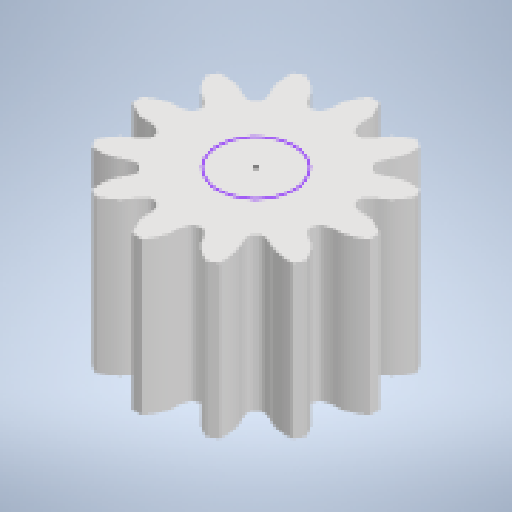
# Autodesk Inventor part: gear_3
Saved by Autodesk Inventor 2025.2 (Build 292293000, 293)
## iProperties
Created: 2025-03-25
Part Number: gear_3
Material: Generic
Document SubType Name: Modeling
Designer: Admin
Density: 1 g/cm^3
Appearance: Default
Author: Admin
Autodesk Inventor part; units mm, degrees
ref_plane "YZ Plane" through (0, 0, 0) normal (1, 0, 0) x (0, 1, 0)
ref_plane "XZ Plane" through (0, 0, 0) normal (0, 1, 0) x (-1, 0, 0)
ref_plane "XY Plane" through (0, 0, 0) normal (0, 0, 1) x (1, 0, 0)
sketch "Sketch1" plane through (0, 0, 0) normal (0, 1, 0) x (-1, 0, 0)
  arc A0 (0.3103, 6.9931) -> (-0.3103, 6.9931) centre (0, 0) ccw
  spline S0 degree 3 poles (-0.3103, 6.9931) (-0.3386, 6.9508) (-0.3937, 6.8652) (-0.4712, 6.7337) (-0.5433, 6.5992) (-0.6093, 6.4615) (-0.6693, 6.3211) (-0.7218, 6.1777) (-0.7653, 6.0313) (-0.7979, 5.8823) (-0.8227, 5.7311) (-0.8192, 5.5783) (-0.8156, 5.4255) (-0.8404, 5.2744) (-0.873, 5.1254) (-0.906, 5.0145) (-0.9268, 4.9533) (-0.9314, 4.9403) knots 0.009806 0.009806 0.009806 0.009806 0.07852 0.147233 0.215945 0.284657 0.353368 0.422077 0.490783 0.559487 0.628183 0.696834 0.765485 0.834181 0.902886 0.971592 0.990196 0.990196 0.990196 0.990196
  arc A1 (-1.2026, 4.6913) -> (-0.9314, 4.9403) centre (-1.2995, 5.0691) ccw
  arc A2 (-1.2026, 4.6913) -> (-1.3041, 4.6641) centre (0, 0) ccw
  arc A3 (-1.6636, 4.7441) -> (-1.3041, 4.6641) centre (-1.4091, 5.0397) ccw
  spline S1 degree 3 poles (-1.6636, 4.7441) (-1.674, 4.7531) (-1.7227, 4.7957) (-1.8066, 4.8752) (-1.9094, 4.988) (-2.0064, 5.1065) (-2.0798, 5.2406) (-2.1531, 5.3747) (-2.2501, 5.4932) (-2.3529, 5.6059) (-2.4638, 5.711) (-2.5809, 5.8089) (-2.7031, 5.9005) (-2.8291, 5.9867) (-2.9588, 6.0672) (-3.0917, 6.1423) (-3.1821, 6.1889) (-3.2278, 6.2114) knots 0.009805 0.009805 0.009805 0.009805 0.028409 0.097115 0.165819 0.234515 0.303166 0.371817 0.440513 0.509218 0.577924 0.646632 0.715343 0.784055 0.852768 0.921481 0.990194 0.990194 0.990194 0.990194
  arc A4 (-3.2278, 6.2114) -> (-3.7653, 5.901) centre (0, 0) ccw
  spline S2 degree 3 poles (-3.7653, 5.901) (-3.7687, 5.8503) (-3.7736, 5.7486) (-3.775, 5.596) (-3.7701, 5.4434) (-3.7584, 5.2912) (-3.7401, 5.1396) (-3.7139, 4.9892) (-3.6784, 4.8406) (-3.6322, 4.6952) (-3.578, 4.552) (-3.4986, 4.4214) (-3.4191, 4.2908) (-3.365, 4.1476) (-3.3188, 4.0022) (-3.2919, 3.8897) (-3.2793, 3.8263) (-3.2767, 3.8128) knots 0.009806 0.009806 0.009806 0.009806 0.07852 0.147233 0.215945 0.284657 0.353368 0.422077 0.490783 0.559487 0.628183 0.696834 0.765485 0.834181 0.902886 0.971592 0.990196 0.990196 0.990196 0.990196
  arc A5 (-3.3872, 3.4615) -> (-3.2767, 3.8128) centre (-3.6599, 3.7402) ccw
  arc A6 (-3.3872, 3.4615) -> (-3.4615, 3.3872) centre (0, 0) ccw
  arc A7 (-3.8128, 3.2767) -> (-3.4615, 3.3872) centre (-3.7402, 3.6599) ccw
  spline S3 degree 3 poles (-3.8128, 3.2767) (-3.8263, 3.2793) (-3.8897, 3.2919) (-4.0022, 3.3188) (-4.1476, 3.365) (-4.2908, 3.4191) (-4.4214, 3.4986) (-4.552, 3.578) (-4.6952, 3.6322) (-4.8406, 3.6784) (-4.9892, 3.7139) (-5.1396, 3.7401) (-5.2912, 3.7584) (-5.4434, 3.7701) (-5.596, 3.775) (-5.7486, 3.7736) (-5.8503, 3.7687) (-5.901, 3.7653) knots 0.009805 0.009805 0.009805 0.009805 0.028409 0.097115 0.165819 0.234515 0.303166 0.371817 0.440513 0.509218 0.577924 0.646632 0.715343 0.784055 0.852768 0.921481 0.990194 0.990194 0.990194 0.990194
  arc A8 (-5.901, 3.7653) -> (-6.2114, 3.2278) centre (0, 0) ccw
  spline S4 degree 3 poles (-6.2114, 3.2278) (-6.1889, 3.1821) (-6.1423, 3.0917) (-6.0672, 2.9588) (-5.9867, 2.8291) (-5.9005, 2.7031) (-5.8089, 2.5809) (-5.711, 2.4638) (-5.6059, 2.3529) (-5.4932, 2.2501) (-5.3747, 2.1531) (-5.2406, 2.0798) (-5.1065, 2.0064) (-4.988, 1.9094) (-4.8752, 1.8066) (-4.7957, 1.7227) (-4.7531, 1.674) (-4.7441, 1.6636) knots 0.009806 0.009806 0.009806 0.009806 0.07852 0.147233 0.215945 0.284657 0.353368 0.422077 0.490783 0.559487 0.628183 0.696834 0.765485 0.834181 0.902886 0.971592 0.990196 0.990196 0.990196 0.990196
  arc A9 (-4.6641, 1.3041) -> (-4.7441, 1.6636) centre (-5.0397, 1.4091) ccw
  arc A10 (-4.6641, 1.3041) -> (-4.6913, 1.2026) centre (0, 0) ccw
  arc A11 (-4.9403, 0.9314) -> (-4.6913, 1.2026) centre (-5.0691, 1.2995) ccw
  spline S5 degree 3 poles (-4.9403, 0.9314) (-4.9533, 0.9268) (-5.0145, 0.906) (-5.1254, 0.873) (-5.2744, 0.8404) (-5.4255, 0.8156) (-5.5783, 0.8192) (-5.7311, 0.8227) (-5.8823, 0.7979) (-6.0313, 0.7653) (-6.1777, 0.7218) (-6.3211, 0.6693) (-6.4615, 0.6093) (-6.5992, 0.5433) (-6.7337, 0.4712) (-6.8652, 0.3937) (-6.9508, 0.3386) (-6.9931, 0.3103) knots 0.009805 0.009805 0.009805 0.009805 0.028409 0.097115 0.165819 0.234515 0.303166 0.371817 0.440513 0.509218 0.577924 0.646632 0.715343 0.784055 0.852768 0.921481 0.990194 0.990194 0.990194 0.990194
  arc A12 (-6.9931, 0.3103) -> (-6.9931, -0.3103) centre (0, 0) ccw
  spline S6 degree 3 poles (-6.9931, -0.3103) (-6.9508, -0.3386) (-6.8652, -0.3937) (-6.7337, -0.4712) (-6.5992, -0.5433) (-6.4615, -0.6093) (-6.3211, -0.6693) (-6.1777, -0.7218) (-6.0313, -0.7653) (-5.8823, -0.7979) (-5.7311, -0.8227) (-5.5783, -0.8192) (-5.4255, -0.8156) (-5.2744, -0.8404) (-5.1254, -0.873) (-5.0145, -0.906) (-4.9533, -0.9268) (-4.9403, -0.9314) knots 0.009806 0.009806 0.009806 0.009806 0.07852 0.147233 0.215945 0.284657 0.353368 0.422077 0.490783 0.559487 0.628183 0.696834 0.765485 0.834181 0.902886 0.971592 0.990196 0.990196 0.990196 0.990196
  arc A13 (-4.6913, -1.2026) -> (-4.9403, -0.9314) centre (-5.0691, -1.2995) ccw
  arc A14 (-4.6913, -1.2026) -> (-4.6641, -1.3041) centre (0, 0) ccw
  arc A15 (-4.7441, -1.6636) -> (-4.6641, -1.3041) centre (-5.0397, -1.4091) ccw
  spline S7 degree 3 poles (-4.7441, -1.6636) (-4.7531, -1.674) (-4.7957, -1.7227) (-4.8752, -1.8066) (-4.988, -1.9094) (-5.1065, -2.0064) (-5.2406, -2.0798) (-5.3747, -2.1531) (-5.4932, -2.2501) (-5.6059, -2.3529) (-5.711, -2.4638) (-5.8089, -2.5809) (-5.9005, -2.7031) (-5.9867, -2.8291) (-6.0672, -2.9588) (-6.1423, -3.0917) (-6.1889, -3.1821) (-6.2114, -3.2278) knots 0.009805 0.009805 0.009805 0.009805 0.028409 0.097115 0.165819 0.234515 0.303166 0.371817 0.440513 0.509218 0.577924 0.646632 0.715343 0.784055 0.852768 0.921481 0.990194 0.990194 0.990194 0.990194
  arc A16 (-6.2114, -3.2278) -> (-5.901, -3.7653) centre (0, 0) ccw
  spline S8 degree 3 poles (-5.901, -3.7653) (-5.8503, -3.7687) (-5.7486, -3.7736) (-5.596, -3.775) (-5.4434, -3.7701) (-5.2912, -3.7584) (-5.1396, -3.7401) (-4.9892, -3.7139) (-4.8406, -3.6784) (-4.6952, -3.6322) (-4.552, -3.578) (-4.4214, -3.4986) (-4.2908, -3.4191) (-4.1476, -3.365) (-4.0022, -3.3188) (-3.8897, -3.2919) (-3.8263, -3.2793) (-3.8128, -3.2767) knots 0.009806 0.009806 0.009806 0.009806 0.07852 0.147233 0.215945 0.284657 0.353368 0.422077 0.490783 0.559487 0.628183 0.696834 0.765485 0.834181 0.902886 0.971592 0.990196 0.990196 0.990196 0.990196
  arc A17 (-3.4615, -3.3872) -> (-3.8128, -3.2767) centre (-3.7402, -3.6599) ccw
  arc A18 (-3.4615, -3.3872) -> (-3.3872, -3.4615) centre (0, 0) ccw
  arc A19 (-3.2767, -3.8128) -> (-3.3872, -3.4615) centre (-3.6599, -3.7402) ccw
  spline S9 degree 3 poles (-3.2767, -3.8128) (-3.2793, -3.8263) (-3.2919, -3.8897) (-3.3188, -4.0022) (-3.365, -4.1476) (-3.4191, -4.2908) (-3.4986, -4.4214) (-3.578, -4.552) (-3.6322, -4.6952) (-3.6784, -4.8406) (-3.7139, -4.9892) (-3.7401, -5.1396) (-3.7584, -5.2912) (-3.7701, -5.4434) (-3.775, -5.596) (-3.7736, -5.7486) (-3.7687, -5.8503) (-3.7653, -5.901) knots 0.009805 0.009805 0.009805 0.009805 0.028409 0.097115 0.165819 0.234515 0.303166 0.371817 0.440513 0.509218 0.577924 0.646632 0.715343 0.784055 0.852768 0.921481 0.990194 0.990194 0.990194 0.990194
  arc A20 (-3.7653, -5.901) -> (-3.2278, -6.2114) centre (0, 0) ccw
  spline S10 degree 3 poles (-3.2278, -6.2114) (-3.1821, -6.1889) (-3.0917, -6.1423) (-2.9588, -6.0672) (-2.8291, -5.9867) (-2.7031, -5.9005) (-2.5809, -5.8089) (-2.4638, -5.711) (-2.3529, -5.6059) (-2.2501, -5.4932) (-2.1531, -5.3747) (-2.0798, -5.2406) (-2.0064, -5.1065) (-1.9094, -4.988) (-1.8066, -4.8752) (-1.7227, -4.7957) (-1.674, -4.7531) (-1.6636, -4.7441) knots 0.009806 0.009806 0.009806 0.009806 0.07852 0.147233 0.215945 0.284657 0.353368 0.422077 0.490783 0.559487 0.628183 0.696834 0.765485 0.834181 0.902886 0.971592 0.990196 0.990196 0.990196 0.990196
  arc A21 (-1.3041, -4.6641) -> (-1.6636, -4.7441) centre (-1.4091, -5.0397) ccw
  arc A22 (-1.3041, -4.6641) -> (-1.2026, -4.6913) centre (0, 0) ccw
  arc A23 (-0.9314, -4.9403) -> (-1.2026, -4.6913) centre (-1.2995, -5.0691) ccw
  spline S11 degree 3 poles (-0.9314, -4.9403) (-0.9268, -4.9533) (-0.906, -5.0145) (-0.873, -5.1254) (-0.8404, -5.2744) (-0.8156, -5.4255) (-0.8192, -5.5783) (-0.8227, -5.7311) (-0.7979, -5.8823) (-0.7653, -6.0313) (-0.7218, -6.1777) (-0.6693, -6.3211) (-0.6093, -6.4615) (-0.5433, -6.5992) (-0.4712, -6.7337) (-0.3937, -6.8652) (-0.3386, -6.9508) (-0.3103, -6.9931) knots 0.009805 0.009805 0.009805 0.009805 0.028409 0.097115 0.165819 0.234515 0.303166 0.371817 0.440513 0.509218 0.577924 0.646632 0.715343 0.784055 0.852768 0.921481 0.990194 0.990194 0.990194 0.990194
  arc A24 (-0.3103, -6.9931) -> (0.3103, -6.9931) centre (0, 0) ccw
  spline S12 degree 3 poles (0.3103, -6.9931) (0.3386, -6.9508) (0.3937, -6.8652) (0.4712, -6.7337) (0.5433, -6.5992) (0.6093, -6.4615) (0.6693, -6.3211) (0.7218, -6.1777) (0.7653, -6.0313) (0.7979, -5.8823) (0.8227, -5.7311) (0.8192, -5.5783) (0.8156, -5.4255) (0.8404, -5.2744) (0.873, -5.1254) (0.906, -5.0145) (0.9268, -4.9533) (0.9314, -4.9403) knots 0.009806 0.009806 0.009806 0.009806 0.07852 0.147233 0.215945 0.284657 0.353368 0.422077 0.490783 0.559487 0.628183 0.696834 0.765485 0.834181 0.902886 0.971592 0.990196 0.990196 0.990196 0.990196
  arc A25 (1.2026, -4.6913) -> (0.9314, -4.9403) centre (1.2995, -5.0691) ccw
  arc A26 (1.2026, -4.6913) -> (1.3041, -4.6641) centre (0, 0) ccw
  arc A27 (1.6636, -4.7441) -> (1.3041, -4.6641) centre (1.4091, -5.0397) ccw
  spline S13 degree 3 poles (1.6636, -4.7441) (1.674, -4.7531) (1.7227, -4.7957) (1.8066, -4.8752) (1.9094, -4.988) (2.0064, -5.1065) (2.0798, -5.2406) (2.1531, -5.3747) (2.2501, -5.4932) (2.3529, -5.6059) (2.4638, -5.711) (2.5809, -5.8089) (2.7031, -5.9005) (2.8291, -5.9867) (2.9588, -6.0672) (3.0917, -6.1423) (3.1821, -6.1889) (3.2278, -6.2114) knots 0.009805 0.009805 0.009805 0.009805 0.028409 0.097115 0.165819 0.234515 0.303166 0.371817 0.440513 0.509218 0.577924 0.646632 0.715343 0.784055 0.852768 0.921481 0.990194 0.990194 0.990194 0.990194
  arc A28 (3.2278, -6.2114) -> (3.7653, -5.901) centre (0, 0) ccw
  spline S14 degree 3 poles (3.7653, -5.901) (3.7687, -5.8503) (3.7736, -5.7486) (3.775, -5.596) (3.7701, -5.4434) (3.7584, -5.2912) (3.7401, -5.1396) (3.7139, -4.9892) (3.6784, -4.8406) (3.6322, -4.6952) (3.578, -4.552) (3.4986, -4.4214) (3.4191, -4.2908) (3.365, -4.1476) (3.3188, -4.0022) (3.2919, -3.8897) (3.2793, -3.8263) (3.2767, -3.8128) knots 0.009806 0.009806 0.009806 0.009806 0.07852 0.147233 0.215945 0.284657 0.353368 0.422077 0.490783 0.559487 0.628183 0.696834 0.765485 0.834181 0.902886 0.971592 0.990196 0.990196 0.990196 0.990196
  arc A29 (3.3872, -3.4615) -> (3.2767, -3.8128) centre (3.6599, -3.7402) ccw
  arc A30 (3.3872, -3.4615) -> (3.4615, -3.3872) centre (0, 0) ccw
  arc A31 (3.8128, -3.2767) -> (3.4615, -3.3872) centre (3.7402, -3.6599) ccw
  spline S15 degree 3 poles (3.8128, -3.2767) (3.8263, -3.2793) (3.8897, -3.2919) (4.0022, -3.3188) (4.1476, -3.365) (4.2908, -3.4191) (4.4214, -3.4986) (4.552, -3.578) (4.6952, -3.6322) (4.8406, -3.6784) (4.9892, -3.7139) (5.1396, -3.7401) (5.2912, -3.7584) (5.4434, -3.7701) (5.596, -3.775) (5.7486, -3.7736) (5.8503, -3.7687) (5.901, -3.7653) knots 0.009805 0.009805 0.009805 0.009805 0.028409 0.097115 0.165819 0.234515 0.303166 0.371817 0.440513 0.509218 0.577924 0.646632 0.715343 0.784055 0.852768 0.921481 0.990194 0.990194 0.990194 0.990194
  arc A32 (5.901, -3.7653) -> (6.2114, -3.2278) centre (0, 0) ccw
  spline S16 degree 3 poles (6.2114, -3.2278) (6.1889, -3.1821) (6.1423, -3.0917) (6.0672, -2.9588) (5.9867, -2.8291) (5.9005, -2.7031) (5.8089, -2.5809) (5.711, -2.4638) (5.6059, -2.3529) (5.4932, -2.2501) (5.3747, -2.1531) (5.2406, -2.0798) (5.1065, -2.0064) (4.988, -1.9094) (4.8752, -1.8066) (4.7957, -1.7227) (4.7531, -1.674) (4.7441, -1.6636) knots 0.009806 0.009806 0.009806 0.009806 0.07852 0.147233 0.215945 0.284657 0.353368 0.422077 0.490783 0.559487 0.628183 0.696834 0.765485 0.834181 0.902886 0.971592 0.990196 0.990196 0.990196 0.990196
  arc A33 (4.6641, -1.3041) -> (4.7441, -1.6636) centre (5.0397, -1.4091) ccw
  arc A34 (4.6641, -1.3041) -> (4.6913, -1.2026) centre (0, 0) ccw
  arc A35 (4.9403, -0.9314) -> (4.6913, -1.2026) centre (5.0691, -1.2995) ccw
  spline S17 degree 3 poles (4.9403, -0.9314) (4.9533, -0.9268) (5.0145, -0.906) (5.1254, -0.873) (5.2744, -0.8404) (5.4255, -0.8156) (5.5783, -0.8192) (5.7311, -0.8227) (5.8823, -0.7979) (6.0313, -0.7653) (6.1777, -0.7218) (6.3211, -0.6693) (6.4615, -0.6093) (6.5992, -0.5433) (6.7337, -0.4712) (6.8652, -0.3937) (6.9508, -0.3386) (6.9931, -0.3103) knots 0.009805 0.009805 0.009805 0.009805 0.028409 0.097115 0.165819 0.234515 0.303166 0.371817 0.440513 0.509218 0.577924 0.646632 0.715343 0.784055 0.852768 0.921481 0.990194 0.990194 0.990194 0.990194
  arc A36 (6.9931, -0.3103) -> (6.9931, 0.3103) centre (0, 0) ccw
  spline S18 degree 3 poles (6.9931, 0.3103) (6.9508, 0.3386) (6.8652, 0.3937) (6.7337, 0.4712) (6.5992, 0.5433) (6.4615, 0.6093) (6.3211, 0.6693) (6.1777, 0.7218) (6.0313, 0.7653) (5.8823, 0.7979) (5.7311, 0.8227) (5.5783, 0.8192) (5.4255, 0.8156) (5.2744, 0.8404) (5.1254, 0.873) (5.0145, 0.906) (4.9533, 0.9268) (4.9403, 0.9314) knots 0.009806 0.009806 0.009806 0.009806 0.07852 0.147233 0.215945 0.284657 0.353368 0.422077 0.490783 0.559487 0.628183 0.696834 0.765485 0.834181 0.902886 0.971592 0.990196 0.990196 0.990196 0.990196
  arc A37 (4.6913, 1.2026) -> (4.9403, 0.9314) centre (5.0691, 1.2995) ccw
  arc A38 (4.6913, 1.2026) -> (4.6641, 1.3041) centre (0, 0) ccw
  arc A39 (4.7441, 1.6636) -> (4.6641, 1.3041) centre (5.0397, 1.4091) ccw
  spline S19 degree 3 poles (4.7441, 1.6636) (4.7531, 1.674) (4.7957, 1.7227) (4.8752, 1.8066) (4.988, 1.9094) (5.1065, 2.0064) (5.2406, 2.0798) (5.3747, 2.1531) (5.4932, 2.2501) (5.6059, 2.3529) (5.711, 2.4638) (5.8089, 2.5809) (5.9005, 2.7031) (5.9867, 2.8291) (6.0672, 2.9588) (6.1423, 3.0917) (6.1889, 3.1821) (6.2114, 3.2278) knots 0.009805 0.009805 0.009805 0.009805 0.028409 0.097115 0.165819 0.234515 0.303166 0.371817 0.440513 0.509218 0.577924 0.646632 0.715343 0.784055 0.852768 0.921481 0.990194 0.990194 0.990194 0.990194
  arc A40 (6.2114, 3.2278) -> (5.901, 3.7653) centre (0, 0) ccw
  spline S20 degree 3 poles (5.901, 3.7653) (5.8503, 3.7687) (5.7486, 3.7736) (5.596, 3.775) (5.4434, 3.7701) (5.2912, 3.7584) (5.1396, 3.7401) (4.9892, 3.7139) (4.8406, 3.6784) (4.6952, 3.6322) (4.552, 3.578) (4.4214, 3.4986) (4.2908, 3.4191) (4.1476, 3.365) (4.0022, 3.3188) (3.8897, 3.2919) (3.8263, 3.2793) (3.8128, 3.2767) knots 0.009806 0.009806 0.009806 0.009806 0.07852 0.147233 0.215945 0.284657 0.353368 0.422077 0.490783 0.559487 0.628183 0.696834 0.765485 0.834181 0.902886 0.971592 0.990196 0.990196 0.990196 0.990196
  arc A41 (3.4615, 3.3872) -> (3.8128, 3.2767) centre (3.7402, 3.6599) ccw
  arc A42 (3.4615, 3.3872) -> (3.3872, 3.4615) centre (0, 0) ccw
  arc A43 (3.2767, 3.8128) -> (3.3872, 3.4615) centre (3.6599, 3.7402) ccw
  spline S21 degree 3 poles (3.2767, 3.8128) (3.2793, 3.8263) (3.2919, 3.8897) (3.3188, 4.0022) (3.365, 4.1476) (3.4191, 4.2908) (3.4986, 4.4214) (3.578, 4.552) (3.6322, 4.6952) (3.6784, 4.8406) (3.7139, 4.9892) (3.7401, 5.1396) (3.7584, 5.2912) (3.7701, 5.4434) (3.775, 5.596) (3.7736, 5.7486) (3.7687, 5.8503) (3.7653, 5.901) knots 0.009805 0.009805 0.009805 0.009805 0.028409 0.097115 0.165819 0.234515 0.303166 0.371817 0.440513 0.509218 0.577924 0.646632 0.715343 0.784055 0.852768 0.921481 0.990194 0.990194 0.990194 0.990194
  arc A44 (3.7653, 5.901) -> (3.2278, 6.2114) centre (0, 0) ccw
  spline S22 degree 3 poles (3.2278, 6.2114) (3.1821, 6.1889) (3.0917, 6.1423) (2.9588, 6.0672) (2.8291, 5.9867) (2.7031, 5.9005) (2.5809, 5.8089) (2.4638, 5.711) (2.3529, 5.6059) (2.2501, 5.4932) (2.1531, 5.3747) (2.0798, 5.2406) (2.0064, 5.1065) (1.9094, 4.988) (1.8066, 4.8752) (1.7227, 4.7957) (1.674, 4.7531) (1.6636, 4.7441) knots 0.009806 0.009806 0.009806 0.009806 0.07852 0.147233 0.215945 0.284657 0.353368 0.422077 0.490783 0.559487 0.628183 0.696834 0.765485 0.834181 0.902886 0.971592 0.990196 0.990196 0.990196 0.990196
  arc A45 (1.3041, 4.6641) -> (1.6636, 4.7441) centre (1.4091, 5.0397) ccw
  arc A46 (1.3041, 4.6641) -> (1.2026, 4.6913) centre (0, 0) ccw
  arc A47 (0.9314, 4.9403) -> (1.2026, 4.6913) centre (1.2995, 5.0691) ccw
  spline S23 degree 3 poles (0.9314, 4.9403) (0.9268, 4.9533) (0.906, 5.0145) (0.873, 5.1254) (0.8404, 5.2744) (0.8156, 5.4255) (0.8192, 5.5783) (0.8227, 5.7311) (0.7979, 5.8823) (0.7653, 6.0313) (0.7218, 6.1777) (0.6693, 6.3211) (0.6093, 6.4615) (0.5433, 6.5992) (0.4712, 6.7337) (0.3937, 6.8652) (0.3386, 6.9508) (0.3103, 6.9931) knots 0.009805 0.009805 0.009805 0.009805 0.028409 0.097115 0.165819 0.234515 0.303166 0.371817 0.440513 0.509218 0.577924 0.646632 0.715343 0.784055 0.852768 0.921481 0.990194 0.990194 0.990194 0.990194
  circle A48 centre (0, 0) radius 2.5
  dimension "d2" = 5
  constraints: 96 point on circle, 49 centre point, 1 coincident, 48 other
  measures "d2" diameter of A48
extrude "Extrusion1" add sketch "Sketch1" along normal blind 9 contours S23 A47 A46 A45 S22 A44 S21 A43 A42 A41 S20 A40 S19 A39 A38 A37 S18 A36 S17 A35 A34 A33 S16 A32 S15 A31 A30 A29 S14 A28 S13 A27 A26 A25 S12 A24 S11 A23 A22 A21 S10 A20 S9 A19 A18 A17 S8 A16 S7 A15 A14 A13 S6 A12 S5 A11 A10 A9 S4 A8 S3 A7 A6 A5 S2 A4 S1 A3 A2 A1 S0 A0 | A48
sketch "Sketch3" plane through (0, 9, 0) normal (0, 1, 0) x (1, 0, 0)
  circle A0 centre (0, 0) radius 2.2451
  constraints: 1 centre point, 1 coincident
body "Solid1"
